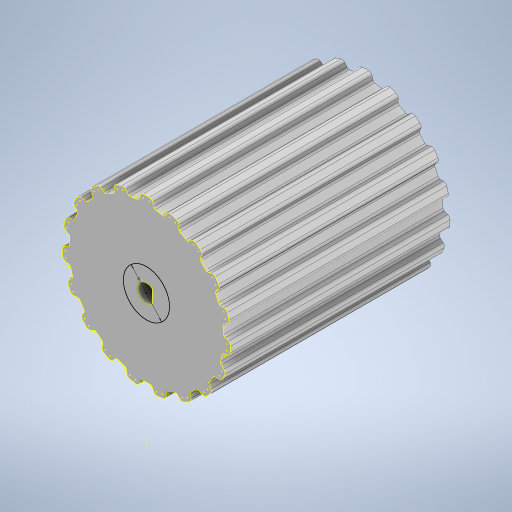
# Autodesk Inventor part: Rodillo2
Saved by Autodesk Inventor 2023 (Build 270158000, 158)
## iProperties
Created: 2023-04-20
Part Number: Rodillo2
Material: Genérico
Document SubType Name: Modeling
Designer: sergi
Density: 1 g/cm^3
Appearance: Valor por defecto
Author: sergi
Autodesk Inventor part; units mm, degrees
ref_plane "YZ Plane" through (0, 0, 0) normal (1, 0, 0) x (0, 1, 0)
ref_plane "XZ Plane" through (0, 0, 0) normal (0, 1, 0) x (-1, 0, 0)
ref_plane "XY Plane" through (0, 0, 0) normal (0, 0, 1) x (1, 0, 0)
sketch "Boceto1" plane through (0, 0, 0) normal (0, 0, 1) x (1, 0, 0)
  circle A0 centre (0, 22.5) radius 9.25 projected
  circle A1 centre (0, 22.5) radius 3.5 projected
  circle A2 centre (0, 27.5) radius 1 projected
  circle A3 centre (0, 17.5) radius 1 projected
  circle A4 centre (0, 22.5) radius 15
  arc A5 (1, 23.618) -> (1, 21.382) centre (0, 22.5) ccw projected
  line L0 (1, 21.382) -> (1, 23.618) projected
  point P0 (0, 0)
  dimension "d0" = 30
  constraints: 1 centre point, 1 coincident
  measures "d0" diameter of A4
extrude "Extrusión1" add sketch "Boceto1" against normal blind 38 contours A0 | A1 | A2 | A3 | A4
sketch "Boceto2" plane through (0, 22.5, -38) normal (0, 0, -1) x (-1, 0, 0)
  circle A0 centre (0, 0) radius 9.5
  point P0 (0, -22.5)
  dimension "d3" = 19
  constraints: 1 centre point
  measures "d3" diameter of A0
extrude "Extrusión2" cut sketch "Boceto2" against normal blind 35
sketch "Boceto3" plane through (0, 22.5, -38) normal (0, 0, -1) x (-1, 0, 0)
  arc A0 (-6.4929, -13.0988) -> (-5.7944, -12.9776) centre (-6.2264, -12.5612) ccw projected
  line L0 (-5.7944, -12.9776) -> (-5.3692, -12.5366) projected
  arc A1 (-4.9514, -12.4358) -> (-5.3692, -12.5366) centre (-5.0812, -12.8142) ccw projected
  line L1 (-4.9514, -12.4358) -> (-3.7309, -12.8548) projected
  arc A2 (-3.463, -13.1909) -> (-3.7309, -12.8548) centre (-3.8608, -13.2331) ccw projected
  line L2 (-3.463, -13.1909) -> (-3.3984, -13.8002) projected
  arc A3 (-3.3984, -13.8002) -> (-2.9217, -14.3248) centre (-2.8018, -13.7369) ccw projected
  arc A4 (-2.9217, -14.3248) -> (-1.8879, -14.4973) centre (0, 0) ccw projected
  arc A5 (-1.8879, -14.4973) -> (-1.2666, -14.1559) centre (-1.8104, -13.9023) ccw projected
  line L3 (-1.2666, -14.1559) -> (-1.0077, -13.6007) projected
  arc A6 (-0.6452, -13.3697) -> (-1.0077, -13.6007) centre (-0.6452, -13.7697) ccw projected
  line L4 (-0.6452, -13.3697) -> (0.6452, -13.3697) projected
  arc A7 (1.0077, -13.6007) -> (0.6452, -13.3697) centre (0.6452, -13.7697) ccw projected
  line L5 (1.0077, -13.6007) -> (1.2666, -14.1559) projected
  arc A8 (1.2666, -14.1559) -> (1.8879, -14.4973) centre (1.8104, -13.9023) ccw projected
  arc A9 (1.8879, -14.4973) -> (2.9217, -14.3248) centre (0, 0) ccw projected
  arc A10 (2.9217, -14.3248) -> (3.3984, -13.8002) centre (2.8018, -13.7369) ccw projected
  line L6 (3.3984, -13.8002) -> (3.463, -13.1909) projected
  arc A11 (3.7309, -12.8548) -> (3.463, -13.1909) centre (3.8608, -13.2331) ccw projected
  line L7 (3.7309, -12.8548) -> (4.9514, -12.4358) projected
  arc A12 (5.3692, -12.5366) -> (4.9514, -12.4358) centre (5.0812, -12.8142) ccw projected
  line L8 (5.3692, -12.5366) -> (5.7944, -12.9776) projected
  arc A13 (5.7944, -12.9776) -> (6.4929, -13.0988) centre (6.2264, -12.5612) ccw projected
  arc A14 (6.4929, -13.0988) -> (7.4146, -12.6) centre (0, 0) ccw projected
  arc A15 (7.4146, -12.6) -> (7.6952, -11.949) centre (7.1103, -12.0829) ccw projected
  line L9 (7.6952, -11.949) -> (7.5585, -11.3518) projected
  arc A16 (7.7027, -10.9469) -> (7.5585, -11.3518) centre (7.9484, -11.2625) ccw projected
  line L10 (7.7027, -10.9469) -> (8.721, -10.1543) projected
  arc A17 (9.1489, -10.1139) -> (8.721, -10.1543) centre (8.9667, -10.47) ccw projected
  line L11 (9.1489, -10.1139) -> (9.6943, -10.393) projected
  arc A18 (9.6943, -10.393) -> (10.3942, -10.2809) centre (9.9676, -9.8589) ccw projected
  arc A19 (10.3942, -10.2809) -> (11.1041, -9.5097) centre (0, 0) ccw projected
  arc A20 (11.1041, -9.5097) -> (11.1581, -8.8029) centre (10.6484, -9.1195) ccw projected
  line L12 (11.1581, -8.8029) -> (10.8349, -8.2825) projected
  arc A21 (10.8398, -7.8527) -> (10.8349, -8.2825) centre (11.1747, -8.0714) ccw projected
  line L13 (10.8398, -7.8527) -> (11.5456, -6.7724) projected
  arc A22 (11.9372, -6.5953) -> (11.5456, -6.7724) centre (11.8804, -6.9912) ccw projected
  line L14 (11.9372, -6.5953) -> (12.5436, -6.6822) projected
  arc A23 (12.5436, -6.6822) -> (13.1692, -6.3488) centre (12.6288, -6.0883) ccw projected
  arc A24 (13.1692, -6.3488) -> (13.5903, -5.389) centre (0, 0) ccw projected
  arc A25 (13.5903, -5.389) -> (13.4118, -4.7029) centre (13.0325, -5.1678) ccw projected
  line L15 (13.4118, -4.7029) -> (12.9371, -4.3156) projected
  arc A26 (12.8022, -3.9075) -> (12.9371, -4.3156) centre (13.19, -4.0057) ccw projected
  line L16 (12.8022, -3.9075) -> (13.119, -2.6566) projected
  arc A27 (13.4319, -2.3619) -> (13.119, -2.6566) centre (13.5068, -2.7548) ccw projected
  line L17 (13.4319, -2.3619) -> (14.0337, -2.2472) projected
  arc A28 (14.0337, -2.2472) -> (14.5171, -1.7288) centre (13.9214, -1.6578) ccw projected
  arc A29 (14.5171, -1.7288) -> (14.6037, -0.6842) centre (0, 0) ccw projected
  arc A30 (14.6037, -0.6842) -> (14.2122, -0.0933) centre (14.0044, -0.6562) ccw projected
  line L18 (14.2122, -0.0933) -> (13.6374, 0.1189) projected
  arc A31 (13.3773, 0.4611) -> (13.6374, 0.1189) centre (13.776, 0.4941) ccw projected
  line L19 (13.3773, 0.4611) -> (13.2708, 1.747) projected
  arc A32 (13.471, 2.1274) -> (13.2708, 1.747) centre (13.6694, 1.7801) ccw projected
  line L20 (13.471, 2.1274) -> (14.003, 2.4313) projected
  arc A33 (14.003, 2.4313) -> (14.2919, 3.0786) centre (13.7054, 2.9523) ccw projected
  arc A34 (14.2919, 3.0786) -> (14.0346, 4.0946) centre (0, 0) ccw projected
  arc A35 (14.0346, 4.0946) -> (13.4724, 4.5264) centre (13.4586, 3.9266) ccw projected
  line L21 (13.4724, 4.5264) -> (12.8599, 4.5405) projected
  arc A36 (12.5028, 4.7797) -> (12.8599, 4.5405) centre (12.8691, 4.9404) ccw projected
  line L22 (12.5028, 4.7797) -> (11.9845, 5.9614) projected
  arc A37 (12.0503, 6.3861) -> (11.9845, 5.9614) centre (12.3508, 6.1221) ccw projected
  line L23 (12.0503, 6.3861) -> (12.4548, 6.8463) projected
  arc A38 (12.4548, 6.8463) -> (12.5179, 7.5524) centre (12.0042, 7.2424) ccw projected
  arc A39 (12.5179, 7.5524) -> (11.9446, 8.4298) centre (0, 0) ccw projected
  arc A40 (11.9446, 8.4298) -> (11.2727, 8.6557) centre (11.4544, 8.0838) ccw projected
  line L24 (11.2727, 8.6557) -> (10.6888, 8.4701) projected
  arc A41 (10.2734, 8.5804) -> (10.6888, 8.4701) centre (10.5677, 8.8513) ccw projected
  line L25 (10.2734, 8.5804) -> (9.3995, 9.5297) projected
  arc A42 (9.3238, 9.9529) -> (9.3995, 9.5297) centre (9.6937, 9.8006) ccw projected
  line L26 (9.3238, 9.9529) -> (9.557, 10.5194) projected
  arc A43 (9.557, 10.5194) -> (9.3874, 11.2077) centre (9.0021, 10.7477) ccw projected
  arc A44 (9.3874, 11.2077) -> (8.5603, 11.8515) centre (0, 0) ccw projected
  arc A45 (8.5603, 11.8515) -> (7.8514, 11.8469) centre (8.209, 11.3651) ccw projected
  line L27 (7.8514, 11.8469) -> (7.3594, 11.4818) projected
  arc A46 (6.9307, 11.4512) -> (7.3594, 11.4818) centre (7.1211, 11.803) ccw projected
  line L28 (6.9307, 11.4512) -> (5.7959, 12.0654) projected
  arc A47 (5.587, 12.441) -> (5.7959, 12.0654) centre (5.9863, 12.4172) ccw projected
  line L29 (5.587, 12.441) -> (5.6235, 13.0526) projected
  arc A48 (5.6235, 13.0526) -> (5.2396, 13.6485) centre (5.0246, 13.0884) ccw projected
  arc A49 (5.2396, 13.6485) -> (4.2483, 13.9889) centre (0, 0) ccw projected
  arc A50 (4.2483, 13.9889) -> (3.5793, 13.7544) centre (4.0739, 13.4147) ccw projected
  line L30 (3.5793, 13.7544) -> (3.2325, 13.2493) projected
  arc A51 (2.837, 13.0812) -> (3.2325, 13.2493) centre (2.9028, 13.4757) ccw projected
  line L31 (2.837, 13.0812) -> (1.5642, 13.2936) projected
  arc A52 (1.2446, 13.581) -> (1.5642, 13.2936) centre (1.63, 13.6881) ccw projected
  line L32 (1.2446, 13.581) -> (1.0807, 14.1713) projected
  arc A53 (1.0807, 14.1713) -> (0.5241, 14.6103) centre (0.5025, 14.0107) ccw projected
  arc A54 (0.5241, 14.6103) -> (-0.5241, 14.6103) centre (0, 0) ccw projected
  arc A55 (-0.5241, 14.6103) -> (-1.0807, 14.1713) centre (-0.5025, 14.0107) ccw projected
  line L33 (-1.0807, 14.1713) -> (-1.2446, 13.581) projected
  arc A56 (-1.5642, 13.2936) -> (-1.2446, 13.581) centre (-1.63, 13.6881) ccw projected
  line L34 (-1.5642, 13.2936) -> (-2.837, 13.0812) projected
  arc A57 (-3.2325, 13.2493) -> (-2.837, 13.0812) centre (-2.9028, 13.4757) ccw projected
  line L35 (-3.2325, 13.2493) -> (-3.5793, 13.7544) projected
  arc A58 (-3.5793, 13.7544) -> (-4.2483, 13.9889) centre (-4.0739, 13.4147) ccw projected
  arc A59 (-4.2483, 13.9889) -> (-5.2396, 13.6485) centre (0, 0) ccw projected
  arc A60 (-5.2396, 13.6485) -> (-5.6235, 13.0526) centre (-5.0246, 13.0884) ccw projected
  line L36 (-5.6235, 13.0526) -> (-5.587, 12.441) projected
  arc A61 (-5.7959, 12.0654) -> (-5.587, 12.441) centre (-5.9863, 12.4172) ccw projected
  line L37 (-5.7959, 12.0654) -> (-6.9307, 11.4512) projected
  arc A62 (-7.3594, 11.4818) -> (-6.9307, 11.4512) centre (-7.1211, 11.803) ccw projected
  line L38 (-7.3594, 11.4818) -> (-7.8514, 11.8469) projected
  arc A63 (-7.8514, 11.8469) -> (-8.5603, 11.8515) centre (-8.209, 11.3651) ccw projected
  arc A64 (-8.5603, 11.8515) -> (-9.3874, 11.2077) centre (0, 0) ccw projected
  arc A65 (-9.3874, 11.2077) -> (-9.557, 10.5194) centre (-9.0021, 10.7477) ccw projected
  line L39 (-9.557, 10.5194) -> (-9.3238, 9.9529) projected
  arc A66 (-9.3995, 9.5297) -> (-9.3238, 9.9529) centre (-9.6937, 9.8006) ccw projected
  line L40 (-9.3995, 9.5297) -> (-10.2734, 8.5804) projected
  arc A67 (-10.6888, 8.4701) -> (-10.2734, 8.5804) centre (-10.5677, 8.8513) ccw projected
  line L41 (-10.6888, 8.4701) -> (-11.2727, 8.6557) projected
  arc A68 (-11.2727, 8.6557) -> (-11.9446, 8.4298) centre (-11.4544, 8.0838) ccw projected
  arc A69 (-11.9446, 8.4298) -> (-12.5179, 7.5524) centre (0, 0) ccw projected
  arc A70 (-12.5179, 7.5524) -> (-12.4548, 6.8463) centre (-12.0042, 7.2424) ccw projected
  line L42 (-12.4548, 6.8463) -> (-12.0503, 6.3861) projected
  arc A71 (-11.9845, 5.9614) -> (-12.0503, 6.3861) centre (-12.3508, 6.1221) ccw projected
  line L43 (-11.9845, 5.9614) -> (-12.5028, 4.7797) projected
  arc A72 (-12.8599, 4.5405) -> (-12.5028, 4.7797) centre (-12.8691, 4.9404) ccw projected
  line L44 (-12.8599, 4.5405) -> (-13.4724, 4.5264) projected
  arc A73 (-13.4724, 4.5264) -> (-14.0346, 4.0946) centre (-13.4586, 3.9266) ccw projected
  arc A74 (-14.0346, 4.0946) -> (-14.2919, 3.0786) centre (0, 0) ccw projected
  arc A75 (-14.2919, 3.0786) -> (-14.003, 2.4313) centre (-13.7054, 2.9523) ccw projected
  line L45 (-14.003, 2.4313) -> (-13.471, 2.1274) projected
  arc A76 (-13.2708, 1.747) -> (-13.471, 2.1274) centre (-13.6694, 1.7801) ccw projected
  line L46 (-13.2708, 1.747) -> (-13.3773, 0.4611) projected
  arc A77 (-13.6374, 0.1189) -> (-13.3773, 0.4611) centre (-13.776, 0.4941) ccw projected
  line L47 (-13.6374, 0.1189) -> (-14.2122, -0.0933) projected
  arc A78 (-14.2122, -0.0933) -> (-14.6037, -0.6842) centre (-14.0044, -0.6562) ccw projected
  arc A79 (-14.6037, -0.6842) -> (-14.5171, -1.7288) centre (0, 0) ccw projected
  arc A80 (-14.5171, -1.7288) -> (-14.0337, -2.2472) centre (-13.9214, -1.6578) ccw projected
  line L48 (-14.0337, -2.2472) -> (-13.4319, -2.3619) projected
  arc A81 (-13.119, -2.6566) -> (-13.4319, -2.3619) centre (-13.5068, -2.7548) ccw projected
  line L49 (-13.119, -2.6566) -> (-12.8022, -3.9075) projected
  arc A82 (-12.9371, -4.3156) -> (-12.8022, -3.9075) centre (-13.19, -4.0057) ccw projected
  line L50 (-12.9371, -4.3156) -> (-13.4118, -4.7029) projected
  arc A83 (-13.4118, -4.7029) -> (-13.5903, -5.389) centre (-13.0325, -5.1678) ccw projected
  arc A84 (-13.5903, -5.389) -> (-13.1692, -6.3488) centre (0, 0) ccw projected
  arc A85 (-13.1692, -6.3488) -> (-12.5436, -6.6822) centre (-12.6288, -6.0883) ccw projected
  line L51 (-12.5436, -6.6822) -> (-11.9372, -6.5953) projected
  arc A86 (-11.5456, -6.7724) -> (-11.9372, -6.5953) centre (-11.8804, -6.9912) ccw projected
  line L52 (-11.5456, -6.7724) -> (-10.8398, -7.8527) projected
  arc A87 (-10.8349, -8.2825) -> (-10.8398, -7.8527) centre (-11.1747, -8.0714) ccw projected
  line L53 (-10.8349, -8.2825) -> (-11.1581, -8.8029) projected
  arc A88 (-11.1581, -8.8029) -> (-11.1041, -9.5097) centre (-10.6484, -9.1195) ccw projected
  arc A89 (-11.1041, -9.5097) -> (-10.3942, -10.2809) centre (0, 0) ccw projected
  arc A90 (-10.3942, -10.2809) -> (-9.6943, -10.393) centre (-9.9676, -9.8589) ccw projected
  line L54 (-9.6943, -10.393) -> (-9.1489, -10.1139) projected
  arc A91 (-8.721, -10.1543) -> (-9.1489, -10.1139) centre (-8.9667, -10.47) ccw projected
  line L55 (-8.721, -10.1543) -> (-7.7027, -10.9469) projected
  arc A92 (-7.5585, -11.3518) -> (-7.7027, -10.9469) centre (-7.9484, -11.2625) ccw projected
  line L56 (-7.5585, -11.3518) -> (-7.6952, -11.949) projected
  arc A93 (-7.6952, -11.949) -> (-7.4146, -12.6) centre (-7.1103, -12.0829) ccw projected
  arc A94 (-7.4146, -12.6) -> (-6.4929, -13.0988) centre (0, 0) ccw projected
  arc A95 (15, 0) -> (-15, 0) centre (0, 0) ccw projected
  circle A96 centre (0, 0) radius 15 projected
  arc A97 (15, 0) -> (-15, 0) centre (0, 0) ccw projected
  arc A98 (16, 0) -> (-16, 0) centre (0, 0) ccw projected
  arc A99 (15, 0) -> (-15, 0) centre (0, 0) ccw projected
  point P0 (0, -22.5)
extrude "Extrusión3" cut sketch "Boceto3" against normal through all
sketch "Boceto5" plane through (0, 0, 0) normal (0, 0, 1) x (1, 0, 0)
  line L0 (7.7027, 11.5531) -> (8.721, 12.3457) projected
  arc A0 (9.1489, 12.3861) -> (8.721, 12.3457) centre (8.9667, 12.03) ccw projected
  line L1 (9.1489, 12.3861) -> (9.6943, 12.107) projected
  arc A1 (9.6943, 12.107) -> (10.3942, 12.2191) centre (9.9676, 12.6411) ccw projected
  arc A2 (10.3942, 12.2191) -> (11.1041, 12.9903) centre (0, 22.5) ccw projected
  arc A3 (11.1041, 12.9903) -> (11.1581, 13.6971) centre (10.6484, 13.3805) ccw projected
  line L2 (11.1581, 13.6971) -> (10.8349, 14.2175) projected
  arc A4 (10.8398, 14.6473) -> (10.8349, 14.2175) centre (11.1747, 14.4286) ccw projected
  line L3 (10.8398, 14.6473) -> (11.5456, 15.7276) projected
  arc A5 (11.9372, 15.9047) -> (11.5456, 15.7276) centre (11.8804, 15.5088) ccw projected
  line L4 (11.9372, 15.9047) -> (12.5436, 15.8178) projected
  arc A6 (12.5436, 15.8178) -> (13.1692, 16.1512) centre (12.6288, 16.4117) ccw projected
  arc A7 (13.1692, 16.1512) -> (13.5903, 17.111) centre (0, 22.5) ccw projected
  arc A8 (13.5903, 17.111) -> (13.4118, 17.7971) centre (13.0325, 17.3322) ccw projected
  line L5 (13.4118, 17.7971) -> (12.9371, 18.1844) projected
  arc A9 (12.8022, 18.5925) -> (12.9371, 18.1844) centre (13.19, 18.4943) ccw projected
  line L6 (12.8022, 18.5925) -> (13.119, 19.8434) projected
  arc A10 (13.4319, 20.1381) -> (13.119, 19.8434) centre (13.5068, 19.7452) ccw projected
  line L7 (13.4319, 20.1381) -> (14.0337, 20.2528) projected
  arc A11 (14.0337, 20.2528) -> (14.5171, 20.7712) centre (13.9214, 20.8422) ccw projected
  arc A12 (14.5171, 20.7712) -> (14.6037, 21.8158) centre (0, 22.5) ccw projected
  arc A13 (14.6037, 21.8158) -> (14.2122, 22.4067) centre (14.0044, 21.8438) ccw projected
  line L8 (14.2122, 22.4067) -> (13.6374, 22.6189) projected
  arc A14 (13.3773, 22.9611) -> (13.6374, 22.6189) centre (13.776, 22.9941) ccw projected
  line L9 (13.3773, 22.9611) -> (13.2708, 24.247) projected
  arc A15 (13.471, 24.6274) -> (13.2708, 24.247) centre (13.6694, 24.2801) ccw projected
  line L10 (13.471, 24.6274) -> (14.003, 24.9313) projected
  arc A16 (14.003, 24.9313) -> (14.2919, 25.5786) centre (13.7054, 25.4523) ccw projected
  arc A17 (14.2919, 25.5786) -> (14.0346, 26.5946) centre (0, 22.5) ccw projected
  arc A18 (14.0346, 26.5946) -> (13.4724, 27.0264) centre (13.4586, 26.4266) ccw projected
  line L11 (13.4724, 27.0264) -> (12.8599, 27.0405) projected
  arc A19 (12.5028, 27.2797) -> (12.8599, 27.0405) centre (12.8691, 27.4404) ccw projected
  line L12 (12.5028, 27.2797) -> (11.9845, 28.4614) projected
  arc A20 (12.0503, 28.8861) -> (11.9845, 28.4614) centre (12.3508, 28.6221) ccw projected
  line L13 (12.0503, 28.8861) -> (12.4548, 29.3463) projected
  arc A21 (12.4548, 29.3463) -> (12.5179, 30.0524) centre (12.0042, 29.7424) ccw projected
  arc A22 (12.5179, 30.0524) -> (11.9446, 30.9298) centre (0, 22.5) ccw projected
  arc A23 (11.9446, 30.9298) -> (11.2727, 31.1557) centre (11.4544, 30.5838) ccw projected
  line L14 (11.2727, 31.1557) -> (10.6888, 30.9701) projected
  arc A24 (10.2734, 31.0804) -> (10.6888, 30.9701) centre (10.5677, 31.3513) ccw projected
  line L15 (10.2734, 31.0804) -> (9.3995, 32.0297) projected
  arc A25 (9.3238, 32.4529) -> (9.3995, 32.0297) centre (9.6937, 32.3006) ccw projected
  line L16 (9.3238, 32.4529) -> (9.557, 33.0194) projected
  arc A26 (9.557, 33.0194) -> (9.3874, 33.7077) centre (9.0021, 33.2477) ccw projected
  arc A27 (9.3874, 33.7077) -> (8.5603, 34.3515) centre (0, 22.5) ccw projected
  arc A28 (8.5603, 34.3515) -> (7.8514, 34.3469) centre (8.209, 33.8651) ccw projected
  line L17 (7.8514, 34.3469) -> (7.3594, 33.9818) projected
  arc A29 (6.9307, 33.9512) -> (7.3594, 33.9818) centre (7.1211, 34.303) ccw projected
  line L18 (6.9307, 33.9512) -> (5.7959, 34.5654) projected
  arc A30 (5.587, 34.941) -> (5.7959, 34.5654) centre (5.9863, 34.9172) ccw projected
  line L19 (5.587, 34.941) -> (5.6235, 35.5526) projected
  arc A31 (5.6235, 35.5526) -> (5.2396, 36.1485) centre (5.0246, 35.5884) ccw projected
  arc A32 (5.2396, 36.1485) -> (4.2483, 36.4889) centre (0, 22.5) ccw projected
  arc A33 (4.2483, 36.4889) -> (3.5793, 36.2544) centre (4.0739, 35.9147) ccw projected
  line L20 (3.5793, 36.2544) -> (3.2325, 35.7493) projected
  arc A34 (2.837, 35.5812) -> (3.2325, 35.7493) centre (2.9028, 35.9757) ccw projected
  line L21 (2.837, 35.5812) -> (1.5642, 35.7936) projected
  arc A35 (1.2446, 36.081) -> (1.5642, 35.7936) centre (1.63, 36.1881) ccw projected
  line L22 (1.2446, 36.081) -> (1.0807, 36.6713) projected
  arc A36 (1.0807, 36.6713) -> (0.5241, 37.1103) centre (0.5025, 36.5107) ccw projected
  arc A37 (0.5241, 37.1103) -> (-0.5241, 37.1103) centre (0, 22.5) ccw projected
  arc A38 (-0.5241, 37.1103) -> (-1.0807, 36.6713) centre (-0.5025, 36.5107) ccw projected
  line L23 (-1.0807, 36.6713) -> (-1.2446, 36.081) projected
  arc A39 (-1.5642, 35.7936) -> (-1.2446, 36.081) centre (-1.63, 36.1881) ccw projected
  line L24 (-1.5642, 35.7936) -> (-2.837, 35.5812) projected
  arc A40 (-3.2325, 35.7493) -> (-2.837, 35.5812) centre (-2.9028, 35.9757) ccw projected
  line L25 (-3.2325, 35.7493) -> (-3.5793, 36.2544) projected
  arc A41 (-3.5793, 36.2544) -> (-4.2483, 36.4889) centre (-4.0739, 35.9147) ccw projected
  arc A42 (-4.2483, 36.4889) -> (-5.2396, 36.1485) centre (0, 22.5) ccw projected
  arc A43 (-5.2396, 36.1485) -> (-5.6235, 35.5526) centre (-5.0246, 35.5884) ccw projected
  line L26 (-5.6235, 35.5526) -> (-5.587, 34.941) projected
  arc A44 (-5.7959, 34.5654) -> (-5.587, 34.941) centre (-5.9863, 34.9172) ccw projected
  line L27 (-5.7959, 34.5654) -> (-6.9307, 33.9512) projected
  arc A45 (-7.3594, 33.9818) -> (-6.9307, 33.9512) centre (-7.1211, 34.303) ccw projected
  line L28 (-7.3594, 33.9818) -> (-7.8514, 34.3469) projected
  arc A46 (-7.8514, 34.3469) -> (-8.5603, 34.3515) centre (-8.209, 33.8651) ccw projected
  arc A47 (-8.5603, 34.3515) -> (-9.3874, 33.7077) centre (0, 22.5) ccw projected
  arc A48 (-9.3874, 33.7077) -> (-9.557, 33.0194) centre (-9.0021, 33.2477) ccw projected
  line L29 (-9.557, 33.0194) -> (-9.3238, 32.4529) projected
  arc A49 (-9.3995, 32.0297) -> (-9.3238, 32.4529) centre (-9.6937, 32.3006) ccw projected
  line L30 (-9.3995, 32.0297) -> (-10.2734, 31.0804) projected
  arc A50 (-10.6888, 30.9701) -> (-10.2734, 31.0804) centre (-10.5677, 31.3513) ccw projected
  line L31 (-10.6888, 30.9701) -> (-11.2727, 31.1557) projected
  arc A51 (-11.2727, 31.1557) -> (-11.9446, 30.9298) centre (-11.4544, 30.5838) ccw projected
  arc A52 (-11.9446, 30.9298) -> (-12.5179, 30.0524) centre (0, 22.5) ccw projected
  arc A53 (-12.5179, 30.0524) -> (-12.4548, 29.3463) centre (-12.0042, 29.7424) ccw projected
  line L32 (-12.4548, 29.3463) -> (-12.0503, 28.8861) projected
  arc A54 (-11.9845, 28.4614) -> (-12.0503, 28.8861) centre (-12.3508, 28.6221) ccw projected
  line L33 (-11.9845, 28.4614) -> (-12.5028, 27.2797) projected
  arc A55 (-12.8599, 27.0405) -> (-12.5028, 27.2797) centre (-12.8691, 27.4404) ccw projected
  line L34 (-12.8599, 27.0405) -> (-13.4724, 27.0264) projected
  arc A56 (-13.4724, 27.0264) -> (-14.0346, 26.5946) centre (-13.4586, 26.4266) ccw projected
  arc A57 (-14.0346, 26.5946) -> (-14.2919, 25.5786) centre (0, 22.5) ccw projected
  arc A58 (-14.2919, 25.5786) -> (-14.003, 24.9313) centre (-13.7054, 25.4523) ccw projected
  line L35 (-14.003, 24.9313) -> (-13.471, 24.6274) projected
  arc A59 (-13.2708, 24.247) -> (-13.471, 24.6274) centre (-13.6694, 24.2801) ccw projected
  line L36 (-13.2708, 24.247) -> (-13.3773, 22.9611) projected
  arc A60 (-13.6374, 22.6189) -> (-13.3773, 22.9611) centre (-13.776, 22.9941) ccw projected
  line L37 (-13.6374, 22.6189) -> (-14.2122, 22.4067) projected
  arc A61 (-14.2122, 22.4067) -> (-14.6037, 21.8158) centre (-14.0044, 21.8438) ccw projected
  arc A62 (-14.6037, 21.8158) -> (-14.5171, 20.7712) centre (0, 22.5) ccw projected
  arc A63 (-14.5171, 20.7712) -> (-14.0337, 20.2528) centre (-13.9214, 20.8422) ccw projected
  line L38 (-14.0337, 20.2528) -> (-13.4319, 20.1381) projected
  arc A64 (-13.119, 19.8434) -> (-13.4319, 20.1381) centre (-13.5068, 19.7452) ccw projected
  line L39 (-13.119, 19.8434) -> (-12.8022, 18.5925) projected
  arc A65 (-12.9371, 18.1844) -> (-12.8022, 18.5925) centre (-13.19, 18.4943) ccw projected
  line L40 (-12.9371, 18.1844) -> (-13.4118, 17.7971) projected
  arc A66 (-13.4118, 17.7971) -> (-13.5903, 17.111) centre (-13.0325, 17.3322) ccw projected
  arc A67 (-13.5903, 17.111) -> (-13.1692, 16.1512) centre (0, 22.5) ccw projected
  arc A68 (-13.1692, 16.1512) -> (-12.5436, 15.8178) centre (-12.6288, 16.4117) ccw projected
  line L41 (-12.5436, 15.8178) -> (-11.9372, 15.9047) projected
  arc A69 (-11.5456, 15.7276) -> (-11.9372, 15.9047) centre (-11.8804, 15.5088) ccw projected
  line L42 (-11.5456, 15.7276) -> (-10.8398, 14.6473) projected
  arc A70 (-10.8349, 14.2175) -> (-10.8398, 14.6473) centre (-11.1747, 14.4286) ccw projected
  line L43 (-10.8349, 14.2175) -> (-11.1581, 13.6971) projected
  arc A71 (-11.1581, 13.6971) -> (-11.1041, 12.9903) centre (-10.6484, 13.3805) ccw projected
  arc A72 (-11.1041, 12.9903) -> (-10.3942, 12.2191) centre (0, 22.5) ccw projected
  arc A73 (-10.3942, 12.2191) -> (-9.6943, 12.107) centre (-9.9676, 12.6411) ccw projected
  line L44 (-9.6943, 12.107) -> (-9.1489, 12.3861) projected
  arc A74 (-8.721, 12.3457) -> (-9.1489, 12.3861) centre (-8.9667, 12.03) ccw projected
  line L45 (-8.721, 12.3457) -> (-7.7027, 11.5531) projected
  arc A75 (-7.5585, 11.1482) -> (-7.7027, 11.5531) centre (-7.9484, 11.2375) ccw projected
  line L46 (-7.5585, 11.1482) -> (-7.6952, 10.551) projected
  arc A76 (-7.6952, 10.551) -> (-7.4146, 9.9) centre (-7.1103, 10.4171) ccw projected
  arc A77 (-7.4146, 9.9) -> (-6.4929, 9.4012) centre (0, 22.5) ccw projected
  arc A78 (-6.4929, 9.4012) -> (-5.7944, 9.5224) centre (-6.2264, 9.9388) ccw projected
  line L47 (-5.7944, 9.5224) -> (-5.3692, 9.9634) projected
  arc A79 (-4.9514, 10.0642) -> (-5.3692, 9.9634) centre (-5.0812, 9.6858) ccw projected
  line L48 (-4.9514, 10.0642) -> (-3.7309, 9.6452) projected
  arc A80 (-3.463, 9.3091) -> (-3.7309, 9.6452) centre (-3.8608, 9.2669) ccw projected
  line L49 (-3.463, 9.3091) -> (-3.3984, 8.6998) projected
  arc A81 (-3.3984, 8.6998) -> (-2.9217, 8.1752) centre (-2.8018, 8.7631) ccw projected
  arc A82 (-2.9217, 8.1752) -> (-1.8879, 8.0027) centre (0, 22.5) ccw projected
  arc A83 (-1.8879, 8.0027) -> (-1.2666, 8.3441) centre (-1.8104, 8.5977) ccw projected
  line L50 (-1.2666, 8.3441) -> (-1.0077, 8.8993) projected
  arc A84 (-0.6452, 9.1303) -> (-1.0077, 8.8993) centre (-0.6452, 8.7303) ccw projected
  line L51 (-0.6452, 9.1303) -> (0.6452, 9.1303) projected
  arc A85 (1.0077, 8.8993) -> (0.6452, 9.1303) centre (0.6452, 8.7303) ccw projected
  line L52 (1.0077, 8.8993) -> (1.2666, 8.3441) projected
  arc A86 (1.2666, 8.3441) -> (1.8879, 8.0027) centre (1.8104, 8.5977) ccw projected
  arc A87 (1.8879, 8.0027) -> (2.9217, 8.1752) centre (0, 22.5) ccw projected
  arc A88 (2.9217, 8.1752) -> (3.3984, 8.6998) centre (2.8018, 8.7631) ccw projected
  line L53 (3.3984, 8.6998) -> (3.463, 9.3091) projected
  arc A89 (3.7309, 9.6452) -> (3.463, 9.3091) centre (3.8608, 9.2669) ccw projected
  line L54 (3.7309, 9.6452) -> (4.9514, 10.0642) projected
  arc A90 (5.3692, 9.9634) -> (4.9514, 10.0642) centre (5.0812, 9.6858) ccw projected
  line L55 (5.3692, 9.9634) -> (5.7944, 9.5224) projected
  arc A91 (5.7944, 9.5224) -> (6.4929, 9.4012) centre (6.2264, 9.9388) ccw projected
  arc A92 (6.4929, 9.4012) -> (7.4146, 9.9) centre (0, 22.5) ccw projected
  arc A93 (7.4146, 9.9) -> (7.6952, 10.551) centre (7.1103, 10.4171) ccw projected
  line L56 (7.6952, 10.551) -> (7.5585, 11.1482) projected
  arc A94 (7.7027, 11.5531) -> (7.5585, 11.1482) centre (7.9484, 11.2375) ccw projected
  line L57 (1, 23.618) -> (1, 21.382) projected
  arc A95 (1, 23.618) -> (1, 21.382) centre (0, 22.5) ccw projected
  circle A96 centre (0, 22.5) radius 4
  point P0 (0, 0)
  dimension "d11" = 8
  constraints: 1 centre point, 1 coincident
  measures "d11" diameter of A96
